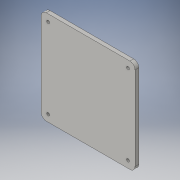
# Autodesk Inventor part: VESA mount
Saved by Autodesk Inventor 2016 (Build 200138000, 138)
## iProperties
Created: 2017-11-13
Part Number: VESA mount
Material: Generic
Document SubType Name: Modeling
Designer: student
Density: 1 g/cm^3
Appearance: Default
Author: student
Autodesk Inventor part; units mm, degrees
ref_plane "YZ Plane" through (0, 0, 0) normal (1, 0, 0) x (0, 1, 0)
ref_plane "XZ Plane" through (0, 0, 0) normal (0, 1, 0) x (-1, 0, 0)
ref_plane "XY Plane" through (0, 0, 0) normal (0, 0, 1) x (1, 0, 0)
sketch "Sketch1" plane through (0, 0, 0) normal (0, 0, 1) x (1, 0, 0)
  line L0 (-58.7375, -58.7375) -> (58.7375, -58.7375)
  line L1 (58.7375, -58.7375) -> (58.7375, 58.7375)
  line L2 (58.7375, 58.7375) -> (-58.7375, 58.7375)
  line L3 (-58.7375, 58.7375) -> (-58.7375, -58.7375)
  circle A0 centre (-50, 50) radius 1.8415
  circle A1 centre (50, 50) radius 1.8415
  circle A2 centre (50, -50) radius 1.8415
  circle A3 centre (-50, -50) radius 1.8415
  line L4 (-50, 50) -> (50, 50)
  line L5 (50, 50) -> (50, -50)
  line L6 (50, -50) -> (-50, -50)
  line L7 (-50, -50) -> (-50, 50)
  point P0 (0, 0)
  point P1 (-51.5938, 0)
  point P2 (0, 50)
  point P3 (-50, 0)
  dimension "d0" = 117.475
  dimension "d1" = 117.475
  dimension "d2" = 3.683
  dimension "d7" = 3.683
  dimension "d11" = 3.683
  dimension "d29" = 100
  dimension "d30" = 100
  dimension "d31" = 100
  dimension "d32" = 3.683
  constraints: 16 end point, 4 centre point, 3 horizontal, 2 horizontal alignment, 2 midpoint, 2 parallel, 2 vertical alignment, 1 perpendicular
  measures "d0" distance of L1.end L2.end
  measures "d1" distance of L0.end L1.end
  measures "d2" diameter of A0
  measures "d7" diameter of A1
  measures "d11" diameter of A2
  measures "d29" distance of L4.end L4.start
  measures "d30" distance of L4.end L5.end
  measures "d31" distance of L5.end L6.end
  measures "d32" diameter of A3
extrude "Extrusion1" add sketch "Sketch1" along normal blind 4.7625 contours L3 L2 L1 L0 | L4 A1 L5 A2 L6 A3 L7 A0
fillet "Fillet1" radius 6.35 4 edges at (58.7375, 58.7375, 2.3813) (-58.7375, 58.7375, 2.3813) (58.7375, -58.7375, 2.3813) (-58.7375, -58.7375, 2.3813)
body "Solid1"
